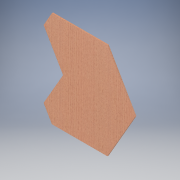
# Autodesk Inventor part: BA015
Saved by Autodesk Inventor 2017 (Build 210142000, 142)
## iProperties
Created: 2018-10-18
Part Number: BA015
Material: Wood (Oak)
Document SubType Name: Modeling
Designer: Dell
Density: 0.76 g/cm^3
Appearance: White Oak - Natural Medium Gloss
Author: Dell
Autodesk Inventor part; units mm, degrees
ref_plane "YZ Plane" through (0, 0, 0) normal (1, 0, 0) x (0, 1, 0)
ref_plane "XZ Plane" through (0, 0, 0) normal (0, 1, 0) x (-1, 0, 0)
ref_plane "XY Plane" through (0, 0, 0) normal (0, 0, 1) x (1, 0, 0)
sketch "Sketch1" plane through (0, 0, 0) normal (0, 0, 1) x (1, 0, 0)
  line L0 (146.05, 252.966) -> (292.1, 0)
  line L1 (292.1, 0) -> (146.05, -252.966)
  line L2 (146.05, -252.966) -> (-146.05, -252.966)
  line L3 (-146.05, -252.966) -> (-292.1, 0)
  line L4 (-292.1, 0) -> (-146.05, 252.966)
  line L5 (-146.05, 252.966) -> (146.05, 252.966)
  point P0 (0, 0)
  point P1 (0, 0)
  dimension "d3" = 584.2
  constraints: 12 end point, 1 coincident, 1 horizontal alignment, 13 other
  measures "d3" distance of L0.end L3.end
extrude "Extrusion1" add sketch "Sketch1" along normal blind 6.35
sketch "Sketch2" plane through (0, 0, 6.35) normal (0, 0, 1) x (1, 0, 0)
  line L0 (-210, 100) -> (-145, 100)
  line L1 (-145, 100) -> (-145, -100)
  line L2 (-145, -100) -> (-210, -100)
  line L3 (-210, -100) -> (-210, 100)
  line L4 (-210, -100) -> (-267.735, 0)
  line L5 (-267.735, 0) -> (-210, 100)
  line L6 (-145, 100) -> (-87.265, 0)
  line L7 (-87.265, 0) -> (-145, -100)
  point P0 (0, 0)
  point P1 (-210, 0)
  dimension "d6" = 145
  dimension "d7" = 65
  dimension "d8" = 200
  dimension "d9" = 30
  dimension "d10" = 30
  dimension "d11" = 30
  constraints: 16 end point, 2 horizontal alignment, 2 parallel, 1 horizontal, 1 midpoint, 1 perpendicular
  measures "d6" distance from line of point (0, 0) L1
  measures "d7" distance of L0.start L0.end
  measures "d8" distance of L2.end L0.start
  measures "d9" angle of L3 L4
  measures "d10" angle of L6 L1
  measures "d11" angle of L1 L7
extrude "Extrusion2" cut sketch "Sketch2" against normal through all
sketch "Sketch3" plane through (0, 0, 6.35) normal (0, 0, 1) x (1, 0, 0)
  line L0 (146.05, 252.966) -> (-146.05, 252.966) construction
  line L1 (0, 252.966) -> (0, -252.966) construction
  line L2 (-146.05, -252.966) -> (146.05, -252.966) construction
  line L3 (-210, 100) -> (-145, 100) projected
  line L4 (-145, 100) -> (-87.265, 0) projected
  line L5 (-87.265, 0) -> (-145, -100) projected
  line L6 (-145, -100) -> (-210, -100) projected
  line L7 (-210, -100) -> (-267.735, 0) projected
  line L8 (-267.735, 0) -> (-210, 100) projected
  line L9 (292.1, 0) -> (146.05, 252.966) construction
  line L10 (146.05, 252.966) -> (-146.05, 252.966) construction
  line L11 (-146.05, 252.966) -> (-292.1, 0) construction
  line L12 (-292.1, 0) -> (-146.05, -252.966) construction
  line L13 (-146.05, -252.966) -> (146.05, -252.966) construction
  line L14 (146.05, -252.966) -> (292.1, 0) construction
  line L15 (210, 100) -> (145, 100)
  line L16 (145, 100) -> (87.265, 0)
  line L17 (87.265, 0) -> (145, -100)
  line L18 (145, -100) -> (210, -100)
  line L19 (210, -100) -> (267.735, 0)
  line L20 (267.735, 0) -> (210, 100)
  point P0 (0, 0)
  constraints: 14 end point, 6 symmetric about line, 2 midpoint
extrude "Extrusion3" cut sketch "Sketch3" against normal through all contours L20 L19 L18 L17 L16 L15
sketch "Sketch4" plane through (0, 0, 6.35) normal (0, 0, 1) x (1, 0, 0)
  line L0 (-145, 100) -> (-210, 100) projected
  line L1 (-145, 100) -> (-189.6825, 177.3923)
  line L2 (-292.1, 0) -> (-146.05, 252.966) projected
  line L3 (-145, -100) -> (-87.265, 0) projected
  line L4 (-145, -100) -> (-189.6825, -177.3923)
  line L5 (-146.05, -252.966) -> (-292.1, 0) projected
  line L6 (145, 100) -> (189.6825, 177.3923)
  line L7 (146.05, 252.966) -> (292.1, 0) projected
  line L8 (145, -100) -> (189.6825, -177.3923)
  line L9 (292.1, 0) -> (146.05, -252.966) projected
  line L10 (87.265, 0) -> (145, 100) projected
  line L11 (145, -100) -> (87.265, 0) projected
  line L12 (-145, 100) -> (-87.265, 0) projected
  point P0 (0, 0)
  constraints: 8 end point, 4 collinear, 4 point on line
extrude "Extrusion4" cut sketch "Sketch4" against normal through all
sketch "Sketch5" plane through (0, 0, 6.35) normal (0, 0, 1) x (1, 0, 0)
  line L0 (87.265, 0) -> (189.6825, 177.3923) projected
  line L1 (189.6825, 177.3923) -> (292.1, 0)
  line L2 (292.1, 0) -> (189.6825, -177.3923)
  line L3 (189.6825, -177.3923) -> (87.265, 0) projected
  line L4 (189.6825, 177.3923) -> (146.05, 252.966) projected
  line L5 (146.05, -252.966) -> (189.6825, -177.3923) projected
  point P0 (0, 0)
  constraints: 4 end point, 2 collinear, 1 horizontal alignment, 1 parallel
extrude "Extrusion5" add sketch "Sketch5" against normal blind 6.35
body "Solid1"
